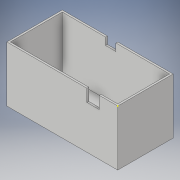
# Autodesk Inventor part: Scannerboxbottom
Saved by Autodesk Inventor 2019 (Build 230136000, 136)
## iProperties
Created: 2018-10-06
Part Number: Scannerboxbottom
Material: Generic
Document SubType Name: Modeling
Designer: paperspace
Density: 1 g/cm^3
Appearance: Default
Author: paperspace
## iProperties of the stored document Scannerboxbottom_3DPrint.ipt
Created: 2018-10-06
Part Number: Scannerboxbottom_3DPrint
Material: Generic
Document SubType Name: Modeling
Designer: paperspace
Density: 1 g/cm^3
Appearance: Default
Author: paperspace
Autodesk Inventor part; units mm, degrees
ref_plane "YZ Plane" through (0, 0, 0) normal (1, 0, 0) x (0, 1, 0)
ref_plane "XZ Plane" through (0, 0, 0) normal (0, 1, 0) x (-1, 0, 0)
ref_plane "XY Plane" through (0, 0, 0) normal (0, 0, 1) x (1, 0, 0)
sketch "Sketch1" plane through (0, 0, 0) normal (0, 1, 0) x (-1, 0, 0)
  line L0 (0, 0) -> (90, 0)
  line L1 (90, 0) -> (90, -45)
  line L2 (90, -45) -> (0, -45)
  line L3 (0, -45) -> (0, 0)
  dimension "d0" = 90
  dimension "d1" = 45
  constraints: 8 end point, 2 parallel, 1 horizontal, 1 perpendicular
  measures "d0" distance of L1.end L2.end
  measures "d1" distance of L0.end L1.end
extrude "Extrusion1" add sketch "Sketch1" along normal blind 45
sketch "Sketch2" plane through (0, 45, 0) normal (0, 1, 0) x (1, 0, 0)
  point P0 (0, 0)
shell "Shell1" thickness 1.5 removed faces 1 at (-30, 45, -15)
sketch "Sketch3" plane through (-90, 0, 0) normal (0, 0, 1) x (1, 0, 0)
  line L0 (75, 35) -> (65, 35)
  line L1 (1.5, 45) -> (88.5, 45) projected
  line L2 (75, 35) -> (65, 35)
  line L3 (65, 35) -> (65, 45)
  line L4 (65, 45) -> (75, 45)
  line L5 (75, 45) -> (75, 35)
  point P0 (90, 0)
  constraints: 10 end point, 2 horizontal, 2 parallel, 1 perpendicular, 1 point on line
extrude "Extrusion2" cut sketch "Sketch3" against normal blind 10
sketch "Sketch4" plane through (0, 0, -45) normal (0, 0, -1) x (-1, 0, 0)
  line L0 (45, 45) -> (53.3446, 45)
  line L1 (53.3446, 45) -> (53.3446, 39.0799)
  line L2 (53.3446, 39.0799) -> (45, 39.0799)
  line L3 (45, 39.0799) -> (45, 45)
  point P0 (0, 0)
  constraints: 8 end point, 2 parallel, 1 horizontal, 1 perpendicular
extrude "Extrusion3" cut sketch "Sketch4" against normal blind 10
body "Solid1"
